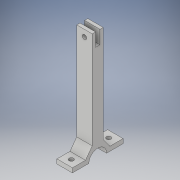
# Autodesk Inventor part: LD_holder_p5
Saved by Autodesk Inventor 2019 (Build 230136000, 136)
## iProperties
Created: 2020-08-30
Part Number: LD_holder_p5
Material: Generic
Document SubType Name: Modeling
Designer: LIU
Density: 1 g/cm^3
Appearance: Default
Author: LIU
Autodesk Inventor part; units mm, degrees
ref_plane "YZ Plane" through (0, 0, 0) normal (1, 0, 0) x (0, 1, 0)
ref_plane "XZ Plane" through (0, 0, 0) normal (0, 1, 0) x (-1, 0, 0)
ref_plane "XY Plane" through (0, 0, 0) normal (0, 0, 1) x (1, 0, 0)
sketch "Sketch1" plane through (0, 0, 0) normal (0, 1, 0) x (-1, 0, 0)
  line L0 (-3.5, 2.5) -> (3.5, 2.5)
  line L1 (3.5, 2.5) -> (3.5, -2.5)
  line L2 (3.5, -2.5) -> (-3.5, -2.5)
  line L3 (-3.5, -2.5) -> (-3.5, 2.5)
  line L4 (-3.5, 2.5) -> (3.5, -2.5) construction
  line L5 (3.5, 2.5) -> (-3.5, -2.5) construction
  point P0 (0, 0)
  dimension "d0" = 5
  dimension "d1" = 7
  constraints: 12 end point, 2 midpoint, 2 parallel, 1 horizontal, 1 perpendicular
  measures "d0" distance of L0.end L1.end
  measures "d1" distance of L0.start L0.end
extrude "Extrusion1" add sketch "Sketch1" along normal blind 50
sketch "Sketch2" plane through (0, 50, 0) normal (0, 1, 0) x (1, 0, 0)
  line L0 (-3.5, -2.5) -> (3.5, -2.5) projected
  line L1 (3.5, -2.5) -> (3.5, 2.5) projected
  line L2 (3.5, 2.5) -> (-3.5, 2.5) projected
  line L3 (-3.5, 2.5) -> (-3.5, -2.5) projected
  line L4 (-3.5, -1) -> (3.5, -1)
  line L5 (3.5, -1) -> (3.5, 1)
  line L6 (3.5, 1) -> (-3.5, 1)
  line L7 (-3.5, 1) -> (-3.5, -1)
  point P0 (0, 0)
  dimension "d4" = 1.5
  dimension "d5" = 1.5
  constraints: 8 end point, 2 parallel, 2 point on line, 1 horizontal, 1 perpendicular
  measures "d4" distance between parallel lines of L2 L6
  measures "d5" distance between parallel lines of L0 L4
extrude "Extrusion2" cut sketch "Sketch2" against normal blind 6 contours L3 L6 L1 L4
sketch "Sketch3" plane through (3.5, 0, -2.5) normal (0, 0, -1) x (-1, 0, 0)
  line L0 (7, 0) -> (7, 50) projected
  line L1 (0, 50) -> (7, 50) projected
  circle A0 centre (3.5, 47) radius 1
  point P0 (3.5, 0)
  dimension "d8" = 2
  dimension "d9" = 3
  dimension "d10" = 3.5
  constraints: 1 centre point
  measures "d8" diameter of A0
  measures "d9" distance from line of L1 A0.centre
  measures "d10" distance from line of L0 A0.centre
extrude "Extrusion3" cut sketch "Sketch3" against normal through all
sketch "Sketch4" plane through (3.5, 0, 2.5) normal (1, 0, 0) x (0, 0, -1)
  line L0 (5, 0) -> (5, 50) projected
  line L1 (0, 0) -> (0, 50) projected
  line L2 (0, 0) -> (5, 0) projected
  circle A0 centre (2.5, 0) radius 4
  line L3 (8.1, 0) -> (-3.1, 0) projected
  dimension "d21" = 8
  constraints: 1 centre point, 1 end point, 1 midpoint
  measures "d21" diameter of A0
extrude "Extrusion4" cut sketch "Sketch4" against normal through all
sketch "Sketch6" plane through (3.5, 44, -1) normal (1, 0, 0) x (0, 0, -1)
  arc A0 (1.5, -40.8775) -> (-3.5, -40.8775) centre (-1, -44) ccw construction
  line L0 (1.5, -40.8775) -> (1.5, 6) projected
  line L1 (-3.5, -40.8775) -> (-3.5, 6) projected
  arc A1 (-3.5, -40.8775) -> (-5, -44) centre (-1, -44) ccw
  line L2 (4.6, -44) -> (-6.6, -44) projected
  line L3 (-15.2174, -44) -> (-5, -44) construction
  arc A2 (1.5, -40.8775) -> (-3.5, -40.8775) centre (-1, -44) ccw
  arc A3 (-5, -44) -> (3, -44) centre (-1, -44) ccw construction
  arc A4 (3, -44) -> (1.5, -40.8775) centre (-1, -44) ccw
  line L4 (-3.5, -37.8775) -> (-6.53, -42)
  line L5 (-1, -58.8) -> (-1, 16.8) projected
  line L6 (-4.4641, -42) -> (-6.53, -42) construction
  line L7 (-12.4641, -42) -> (-12.4641, -44)
  line L8 (-12.4641, -44) -> (-5, -44)
  line L9 (-4.4641, -44) -> (-4.4641, -42) construction
  line L10 (-6.53, -42) -> (-12.4641, -42)
  line L11 (-6.53, -42) -> (-8, -44) construction
  line L12 (-5, -44) -> (17.7359, -44) construction
  line L13 (-5, -44) -> (-4.4641, -44) construction
  line L14 (1.5, -37.8775) -> (4.53, -42)
  line L15 (10.4641, -42) -> (10.4641, -44)
  line L16 (10.4641, -44) -> (3, -44)
  line L17 (4.53, -42) -> (10.4641, -42)
  line L18 (1.5, -37.8775) -> (-3.5, -37.8775)
  dimension "d26" = 3
  dimension "d27" = 3
  dimension "d28" = 8
  dimension "d29" = 2
  constraints: 32 end point, 9 point on circle, 6 point on line, 5 parallel, 4 centre point, 4 symmetric about line, 2 collinear, 2 horizontal, 2 perpendicular, 1 coincident
  measures "d26" distance of L1.start L4.start
  measures "d27" distance of L11.end L3.end
  measures "d28" distance between parallel lines of L7 L9
  measures "d29" distance between parallel lines of L3 L6
extrude "Extrusion5" add sketch "Sketch6" against normal blind 7 contours A2 L5 L18 L0 | L0 L14 L17 L15 L16 L2 A4 | A2 L1 L18 L5 | A1 L2 L8 L7 L10 L4 L1
sketch "Sketch7" plane through (3.5, 2, 11.4641) normal (0, 1, 0) x (1, 0, 0)
  line L0 (-7, 0) -> (-7, 5.9341) projected
  line L1 (0, 0) -> (-7, 0) projected
  circle A0 centre (-3.5, 3) radius 1
  circle A1 centre (-3.5, 19.9282) radius 1
  line L2 (-7, 16.9941) -> (-7, 22.9282) projected
  line L3 (0, 22.9282) -> (-7, 22.9282) projected
  point P0 (-3.5, 11.4641)
  dimension "d32" = 2
  dimension "d33" = 3
  dimension "d34" = 3.5
  dimension "d35" = 3.5
  dimension "d36" = 3
  dimension "d37" = 2
  constraints: 2 centre point
  measures "d32" diameter of A0
  measures "d33" distance from line of L1 A0.centre
  measures "d34" distance from line of L0 A0.centre
  measures "d35" distance from line of L2 A1.centre
  measures "d36" distance from line of L3 A1.centre
  measures "d37" diameter of A1
extrude "Extrusion6" cut sketch "Sketch7" against normal through all
body "Solid1"
